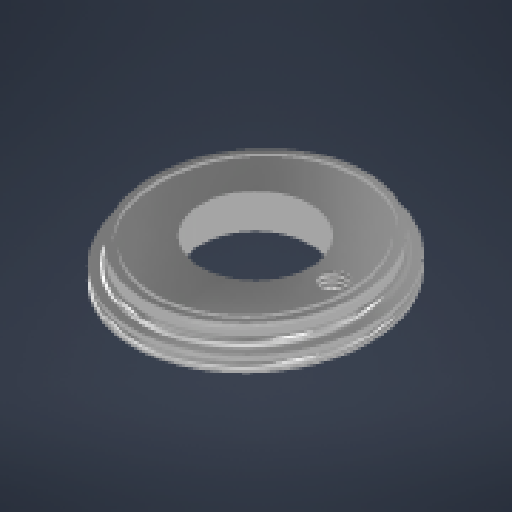
# Autodesk Inventor part: ELIPSE_DRIVE,REV-ENG
Saved by Autodesk Inventor 2026.2 (Build 302298010, 298A)
## iProperties
Created: 2026-03-06
Part Number: ELIPSE_DRIVE,REV-ENG
Material: Steel, 4140, Carb & Flame Harden 58-62 Rc
Document SubType Name: Modeling
Designer: 4aida
Density: 7.86 g/cm^3
Appearance: Chrome - Polished
Author: 4aida
Autodesk Inventor part; units mm, degrees
ref_plane "YZ Plane" through (0, 0, 0) normal (1, 0, 0) x (0, 1, 0)
ref_plane "XZ Plane" through (0, 0, 0) normal (0, 1, 0) x (-1, 0, 0)
ref_plane "XY Plane" through (0, 0, 0) normal (0, 0, 1) x (1, 0, 0)
sketch "Sketch1" plane through (0, 0, 0) normal (0, 1, 0) x (-1, 0, 0)
  ellipse E0 centre (0, 0) end of major axis (0, 16.2) minor radius 15.2
  dimension "d0" = 15.2
  dimension "d1" = 16.2
  constraints: 1 coincident, 2 other
sketch "Sketch2" plane through (0, 0, 0) normal (1, 0, 0) x (0, 1, 0)
  line L0 (-1.1125, 13.7) -> (-1.5, 13.7)
  line L1 (-2.5, 14.7) -> (-2.5, 15.7)
  line L2 (-4.5, 15.7) -> (-4.5, 8.7)
  line L3 (-4.5, 8.7) -> (0, 8.7)
  arc A0 (-2.5, 14.7) -> (-1.5, 13.7) centre (-1.5, 14.7) ccw
  circle A1 centre (-1.25, 14.95) radius 1.25 construction
  line L4 (0, -16.2) -> (0, 16.2) construction
  line L5 (0, 16.2) -> (-3.6965, 16.2) construction
  arc A2 (-4.125, 15.7) -> (-2.875, 15.7) centre (-3.5, 15.7) ccw
  line L6 (-2.5, 15.7) -> (-2.875, 15.7)
  line L7 (-4.125, 15.7) -> (-4.5, 15.7)
  arc A3 (-0.2, 14.1857) -> (-0.283, 14.1415) centre (-0.2, 14.0857) ccw
  arc A4 (-1.1125, 13.7) -> (-0.283, 14.1415) centre (-1.1125, 14.7) ccw
  line L8 (-0.2, 14.1857) -> (0, 14.1857)
  line L9 (0, 12.9357) -> (-0.5, 12.9357)
  line L10 (-0.5, 12.9357) -> (-0.5, 13.4357)
  line L11 (-0.5, 13.4357) -> (0, 13.4357)
  line L12 (0, 8.7) -> (0, 12.9357)
  line L13 (0, 13.4357) -> (0, 14.1857)
  point P0 (0, 0)
  dimension "d2" = 1
  dimension "d3" = 2.5
  dimension "d5" = 2
  dimension "d6" = 5
  dimension "d25" = 1.25
  dimension "d26" = 0.5
  dimension "d27" = 0.375
  dimension "d28" = 0.375
  dimension "d31" = 0.1
  dimension "d33" = 0.01
  dimension "d48" = 0.5
  dimension "d49" = 0.5
  dimension "d50" = 0.75
  dimension "d51" = 0.2
  constraints: 26 end point, 13 perpendicular, 9 tangent, 8 point on circle, 5 centre point, 3 horizontal, 3 point on line, 1 equal radius, 1 horizontal alignment
  measures "d2" radius of A0
  measures "d3" diameter of A1
  measures "d5" distance between parallel lines of L1 L2
  measures "d6" distance between parallel lines of L3 L0
  measures "d25" diameter of A2
  measures "d26" distance between parallel lines of L5 L7
  measures "d27" distance of L1.end L6.end
  measures "d28" distance of L7.start L2.start
  measures "d31" radius of A3
  measures "d48" distance between parallel lines of L11 L9
  measures "d49" distance of L9.start L9.end
  measures "d50" distance from line of L8.end L11
  measures "d51" distance from line of L13 A3.centre
sweep "Sweep1" add profiles "Sketch2" path "Sketch1"
sketch "Sketch7" plane through (0, 0, 0) normal (0, 1, 0) x (-1, 0, 0)
  circle A0 centre (0, 0) radius 7
  spline S0 degree 9 poles (0, 8.7) (-1.2578, 8.7) (-2.5156, 8.4368) (-3.7429, 7.9102) (-4.9102, 7.1162) (-5.9646, 6.0376) (-6.8159, 4.7078) (-7.4054, 3.1985) (-7.9946, 0) (-7.4054, -3.1985) (-6.8159, -4.7078) (-5.9646, -6.0376) (-4.9102, -7.1162) (-3.7429, -7.9102) (-2.5156, -8.4368) (0, -8.9632) (2.5156, -8.4368) (3.7429, -7.9102) (4.9102, -7.1162) (5.9646, -6.0376) (6.8159, -4.7078) (7.4054, -3.1985) (7.9946, 0) (7.4054, 3.1985) (6.8159, 4.7078) (5.9646, 6.0376) (4.9102, 7.1162) (3.7429, 7.9102) (2.5156, 8.4368) (1.2578, 8.7) (0, 8.7) knots 0 0 0 0 0 0 0 0 0 0 0.25 0.25 0.25 0.25 0.25 0.25 0.25 0.5 0.5 0.5 0.5 0.5 0.5 0.5 0.75 0.75 0.75 0.75 0.75 0.75 0.75 1 1 1 1 1 1 1 1 1 1 projected
  dimension "d52" = 14
  constraints: 1 centre point, 1 coincident, 1 other
  measures "d52" diameter of A0
extrude "Extrusion3" add sketch "Sketch7" against normal up to surface (4.5 mm away)
sketch "Sketch8" plane through (0.0167, 0, -0.0005) normal (0, 1, 0) x (1, 0, 0)
  point P0 (-0.0167, -0.0005)
  point P1 (9.9833, -0.0005)
  dimension "d55" = 10
  constraints: 1 horizontal alignment
  measures "d55" distance of point (-0.017, 0) point (9.983, 0)
hole "Hole3" at (10, 0, 0) direction (0, -1, 0) diameter 3.242 depth 5
pattern_circular "Circular Pattern3" count 8 over 360 about axis through (0, 0, 0) along (0, -1, 0) of "Hole3"
equation "\"d28\" = d27"
equation "\"d48\" = d49"
body "Solid1"
